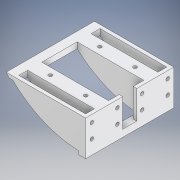
# Autodesk Inventor part: SJ004
Saved by Autodesk Inventor 2017 SP1 (Build 210196100, 196)
## iProperties
Created: 2017-06-03
Part Number: SJ004
Material: ABS Plastic
Document SubType Name: Modeling
Designer: Zach
Density: 1.06 g/cm^3
Appearance: CR White
Author: Zach
Autodesk Inventor part; units mm, degrees
ref_plane "YZ Plane" through (0, 0, 0) normal (1, 0, 0) x (0, 1, 0)
ref_plane "XZ Plane" through (0, 0, 0) normal (0, 1, 0) x (-1, 0, 0)
ref_plane "XY Plane" through (0, 0, 0) normal (0, 0, 1) x (1, 0, 0)
sketch "Sketch3" plane through (0, 0, 0) normal (0, 0, 1) x (1, 0, 0)
  circle A0 centre (0, 130) radius 130 construction
  line L0 (0, 0) -> (0, 10)
  circle A1 centre (0, 130) radius 120 construction
  line L1 (0, 0) -> (0, 50) construction
  line L2 (0, 50) -> (-102.4695, 50) construction
  arc A2 (-102.4695, 50) -> (0, 0) centre (0, 130) ccw
  arc A3 (-89.4427, 50) -> (0, 10) centre (0, 130) ccw
  line L3 (-102.4695, 50) -> (-89.4427, 50)
  dimension "d11" = 260
  dimension "d12" = 10
  dimension "d13" = 10
  dimension "d14" = 50
  constraints: 8 end point, 6 point on circle, 3 centre point, 2 vertical, 1 collinear, 1 concentric, 1 perpendicular, 1 point on line, 1 vertical alignment, 4 other
  measures "d11" diameter of A0
  measures "d12" distance of L0.start L0.end
  measures "d14" distance of L0.start L1.end
extrude "Extrusion2" add sketch "Sketch3" along normal blind 125
sketch "Sketch11" plane through (0, 0, 125) normal (0, 0, 1) x (1, 0, 0)
  line L0 (0, 0) -> (10, 0)
  line L1 (10, 0) -> (10, 10)
  line L2 (10, 10) -> (0, 10)
  line L3 (0, 10) -> (0, 0)
  dimension "d53" = 10
  dimension "d54" = 10
  constraints: 8 end point, 2 parallel, 1 horizontal, 1 perpendicular
  measures "d53" distance of L2.end L1.end
  measures "d54" distance of L1.end L0.end
extrude "Extrusion9" add sketch "Sketch11" against normal blind 125
sketch "Sketch12" plane through (10, 0, 125) normal (1, 0, 0) x (0, 0, -1)
  line L0 (0, 50) -> (0, 0) projected
  line L1 (125, 50) -> (0, 50) projected
  line L2 (0, 0) -> (125, 0)
  line L3 (125, 0) -> (125, 50)
  line L4 (125, 50) -> (0, 50)
  line L5 (0, 50) -> (0, 0)
  constraints: 8 end point, 2 parallel, 1 horizontal, 1 perpendicular
extrude "Extrusion10" add sketch "Sketch12" against normal blind 5
sketch "Sketch13" plane through (0, 0, 125) normal (0, 0, 1) x (1, 0, 0)
  line L0 (5, 10) -> (0, 10) projected
  arc A0 (-89.4427, 50) -> (0, 10) centre (0, 130) ccw projected
  line L1 (-89.4427, 50) -> (-102.4695, 50) projected
  arc A1 (-102.4695, 50) -> (0, 0) centre (0, 130) ccw projected
  line L2 (0, 0) -> (10, 0) projected
  line L3 (10, 0) -> (10, 50) projected
  line L4 (10, 50) -> (5, 50) projected
  line L5 (5, 10) -> (5, 50) projected
  line L6 (-89.4427, 50) -> (-102.4695, 50) projected
  line L7 (-102.4695, 50) -> (10, 50)
  line L8 (10, 0) -> (10, 50) projected
  line L9 (0, 0) -> (10, 0) projected
  line L10 (10, 0) -> (0, 0)
  arc A2 (-102.4695, 50) -> (0, 0) centre (0, 130) ccw
  line L11 (10, 50) -> (10, 0)
  constraints: 6 end point, 3 collinear, 2 point on circle, 1 centre point, 1 concentric
extrude "Extrusion11" add sketch "Sketch13" against normal blind 5 contours L0 A0 L7 L5
sketch "Sketch14" plane through (0, 0, 0) normal (0, 0, -1) x (-1, 0, 0)
  arc A0 (0, 0) -> (102.4695, 50) centre (0, 130) ccw projected
  line L0 (89.4427, 50) -> (102.4695, 50) projected
  arc A1 (0, 10) -> (89.4427, 50) centre (0, 130) ccw projected
  line L1 (-5, 50) -> (89.4427, 50)
  line L2 (-10, 50) -> (102.4695, 50) projected
  line L3 (-5, 10) -> (-5, 50) projected
  line L4 (-5, 10) -> (-5, 50)
  line L5 (0, 10) -> (-5, 10) projected
  line L6 (-5, 10) -> (0, 10)
  arc A2 (0, 10) -> (89.4427, 50) centre (0, 130) ccw projected
  arc A3 (0, 10) -> (89.4427, 50) centre (0, 130) ccw
  line L7 (-10, 0) -> (0, 0) projected
  line L8 (0, 10) -> (-5, 10) projected
  line L9 (-5, 50) -> (-5, 10) projected
  line L10 (-10, 50) -> (-5, 50) projected
  line L11 (-10, 0) -> (-10, 50) projected
  constraints: 6 end point, 3 collinear, 2 point on circle, 1 centre point, 1 concentric
extrude "Extrusion12" add sketch "Sketch14" against normal blind 5 contours A1 L5 L3 L1
sketch "Sketch15" plane through (10, 50, 125) normal (1, 0, 0) x (0, 0, -1)
  line L0 (0, -50) -> (0, 0) construction
  line L1 (0, -50) -> (125, -50) construction
  line L2 (0, 0) -> (20, 0) construction
  line L3 (20, 0) -> (20, -50) construction
  line L4 (20, -50) -> (0, -50) construction
  line L5 (0, -50) -> (0, 0) construction
  line L6 (125, 0) -> (0, 0) construction
  line L7 (37.5, 0) -> (52.5, 0) construction
  line L8 (52.5, 0) -> (52.5, -50) construction
  line L9 (52.5, -50) -> (37.5, -50) construction
  line L10 (37.5, -50) -> (37.5, 0) construction
  line L11 (72.5, 0) -> (87.5, 0) construction
  line L12 (87.5, 0) -> (87.5, -50) construction
  line L13 (87.5, -50) -> (72.5, -50) construction
  line L14 (72.5, -50) -> (72.5, 0) construction
  line L15 (125, -50) -> (125, 0) construction
  line L16 (125, 0) -> (105, 0) construction
  line L17 (105, 0) -> (105, -50) construction
  line L18 (105, -50) -> (125, -50) construction
  line L19 (125, -50) -> (125, 0) construction
  circle A0 centre (8.75, -10) radius 2.5
  circle A1 centre (8.75, -30) radius 2.5
  circle A2 centre (45, -10) radius 2.5
  circle A3 centre (45, -30) radius 2.5
  circle A4 centre (80, -10) radius 2.5
  circle A5 centre (80, -30) radius 2.5
  circle A6 centre (116.25, -10) radius 2.5
  circle A7 centre (116.25, -30) radius 2.5
  dimension "d63" = 20
  dimension "d64" = 15
  dimension "d65" = 20
  dimension "d66" = 15
  dimension "d69" = 5
  dimension "d70" = 5
  dimension "d71" = 5
  dimension "d72" = 5
  dimension "d73" = 5
  dimension "d74" = 5
  dimension "d75" = 5
  dimension "d76" = 5
  dimension "d77" = 8.75
  dimension "d78" = 8.75
  dimension "d79" = 7.5
  dimension "d80" = 7.5
  dimension "d81" = 10
  dimension "d82" = 20
  dimension "d114" = 36.25
  dimension "d115" = 36.25
  constraints: 32 end point, 8 centre point, 8 parallel, 6 horizontal alignment, 6 point on line, 4 horizontal, 4 perpendicular, 4 vertical alignment
  measures "d63" distance of L3.end L4.end
  measures "d64" distance of L12.end L13.end
  measures "d65" distance of L18.end L17.end
  measures "d66" distance between parallel lines of L8 L10
  measures "d69" diameter of A0
  measures "d70" diameter of A1
  measures "d71" diameter of A2
  measures "d72" diameter of A3
  measures "d73" diameter of A4
  measures "d74" diameter of A5
  measures "d75" diameter of A6
  measures "d76" diameter of A7
  measures "d77" distance from line of L19 A6.centre
  measures "d78" distance from line of L0 A0.centre
  measures "d79" distance from line of L10 A2.centre
  measures "d80" distance from line of L14 A4.centre
  measures "d81" distance from line of L6 A0.centre
  measures "d82" distance of A0.centre A1.centre
  measures "d114" distance of A2.centre A0.centre
  measures "d115" distance of A6.centre A4.centre
extrude "Extrusion13" cut sketch "Sketch15" against normal blind 5
sketch "Sketch16" plane through (-102.4695, 50, 125) normal (0, 1, 0) x (1, 0, 0)
  line L0 (112.4695, 125) -> (112.4695, 0) projected
  line L1 (0, 125) -> (0, 0) projected
  line L2 (112.4695, 107.5) -> (0, 107.5)
  line L3 (0, 107.5) -> (0, 87.5)
  line L4 (0, 87.5) -> (112.4695, 87.5)
  line L5 (112.4695, 87.5) -> (112.4695, 107.5)
  line L6 (112.4695, 37.5) -> (0, 37.5)
  line L7 (0, 37.5) -> (0, 17.5)
  line L8 (0, 17.5) -> (112.4695, 17.5)
  line L9 (112.4695, 17.5) -> (112.4695, 37.5)
  line L10 (112.4695, 125) -> (0, 125) projected
  line L11 (0, 0) -> (102.4695, 0) projected
  point P0 (102.4695, 125)
  dimension "d85" = 20
  dimension "d87" = 20
  dimension "d88" = 17.5
  dimension "d89" = 17.5
  constraints: 16 end point, 4 parallel, 4 point on line, 2 horizontal, 2 perpendicular
  measures "d85" distance of L3.end L2.end
  measures "d87" distance of L7.end L6.end
  measures "d88" distance between parallel lines of L10 L2
  measures "d89" distance between parallel lines of L11 L8
extrude "Extrusion14" add sketch "Sketch16" against normal blind 50 contours L0 L4 L1 L2 | L0 L8 L1 L6
sketch "Sketch19" plane through (10, 0, 125) normal (1, 0, 0) x (0, 0, -1)
  line L0 (52.5, 50) -> (72.5, 50)
  line L1 (72.5, 50) -> (72.5, 10)
  line L2 (72.5, 10) -> (52.5, 10)
  line L3 (52.5, 10) -> (52.5, 50)
  line L4 (0, 0) -> (0, 50) projected
  line L5 (125, 50) -> (0, 50) projected
  point P0 (125, 0)
  dimension "d95" = 20
  dimension "d96" = 52.5
  dimension "d97" = 40
  constraints: 8 end point, 2 parallel, 1 horizontal, 1 horizontal alignment, 1 perpendicular, 1 point on line
  measures "d95" distance between parallel lines of L1 L3
  measures "d96" distance between parallel lines of L4 L3
  measures "d97" distance of L2.end L0.start
extrude "Extrusion16" cut sketch "Sketch19" against normal blind 5
sketch "Sketch20" plane through (0, 0, 0) normal (0, 0, -1) x (-1, 0, 0)
  line L0 (0, 0) -> (-10, 0) projected
  arc A0 (0, 0) -> (102.4695, 50) centre (-4.8387, 139.9164) ccw
  line L1 (102.4695, 0) -> (0, 0) projected
  line L2 (0, 0) -> (102.4695, 0)
  line L3 (102.4695, 50) -> (102.4695, 0) projected
  line L4 (102.4695, 0) -> (102.4695, 50)
  line L5 (102.4695, 50) -> (102.4695, 0)
  dimension "d100" = 140
  constraints: 6 end point, 2 collinear, 2 point on circle, 1 centre point, 1 perpendicular
  measures "d100" radius of A0
extrude "Extrusion17" cut sketch "Sketch20" against normal through all
sketch "Sketch21" plane through (-102.4695, 50, 125) normal (0, 1, 0) x (1, 0, 0)
  circle A0 centre (85, 27.5) radius 2.5
  circle A1 centre (35, 27.5) radius 2.5
  circle A2 centre (85, 97.5) radius 2.5
  circle A3 centre (35, 97.5) radius 2.5
  line L0 (102.4695, 17.5) -> (102.4695, 5) projected
  line L1 (13.0268, 17.5) -> (107.4695, 17.5) projected
  line L2 (13.0268, 87.5) -> (107.4695, 87.5) projected
  line L3 (0, 125) -> (0, 0) projected
  dimension "d103" = 5
  dimension "d104" = 5
  dimension "d105" = 5
  dimension "d106" = 5
  dimension "d108" = 50
  dimension "d109" = 10
  dimension "d110" = 10
  dimension "d113" = 35
  constraints: 4 centre point, 2 horizontal alignment, 2 vertical alignment
  measures "d103" diameter of A0
  measures "d104" diameter of A1
  measures "d105" diameter of A2
  measures "d106" diameter of A3
  measures "d108" distance of A0.centre A1.centre
  measures "d109" distance from line of L1 A0.centre
  measures "d110" distance from line of L2 A2.centre
  measures "d113" distance from line of L3 A1.centre
extrude "Extrusion18" cut sketch "Sketch21" against normal through all
sketch "Sketch23" plane through (0, 0, 125) normal (0, 0, 1) x (1, 0, 0)
  line L0 (0, 0) -> (0, 5)
  arc A0 (-98.0733, 45) -> (0, 0) centre (4.8387, 139.9164) ccw
  line L1 (-98.0733, 45) -> (-93.0733, 45)
  arc A1 (-93.0733, 45) -> (0, 5) centre (4.9972, 144.9108) ccw
  arc A2 (-102.4695, 50) -> (0, 0) centre (4.8387, 139.9164) ccw projected
  dimension "d118" = 5
  dimension "d119" = 5
  dimension "d120" = 5
  dimension "d122" = 140
  dimension "d123" = 140
  constraints: 5 point on circle, 4 end point, 2 centre point, 1 horizontal, 1 vertical
  measures "d118" distance of L0.start L0.end
  measures "d119" vertical distance of A2.start L1.start
  measures "d120" distance of L1.start L1.end
  measures "d122" radius of A0
  measures "d123" radius of A1
extrude "Extrusion20" cut sketch "Sketch23" against normal through all
sketch "Sketch24" plane through (-89.4427, 50, 87.5) normal (0, 1, 0) x (1, 0, 0)
  line L0 (0, 82.5) -> (0, 70) projected
  line L1 (89.4427, -37.5) -> (89.4427, 87.5) projected
  line L2 (0, 82.5) -> (89.4427, 82.5)
  line L3 (89.4427, 82.5) -> (89.4427, 69.85)
  line L4 (89.4427, 69.85) -> (0, 69.85)
  line L5 (0, 69.85) -> (0, 82.5)
  line L6 (94.4427, 0) -> (0, 0) projected
  line L7 (89.4427, 50) -> (89.4427, 0) projected
  line L8 (0, 0) -> (89.4427, 0)
  line L9 (89.4427, 0) -> (89.4427, 50)
  line L10 (89.4427, 50) -> (0, 50)
  line L11 (0, 50) -> (0, 0)
  line L12 (0, -32.5) -> (94.4427, -32.5) projected
  line L13 (94.4427, -20) -> (89.4427, -20) projected
  line L14 (0, -32.5) -> (89.4427, -32.5)
  line L15 (89.4427, -32.5) -> (89.4427, -20)
  line L16 (89.4427, -20) -> (0, -20)
  line L17 (0, -20) -> (0, -32.5)
  constraints: 24 end point, 6 parallel, 3 horizontal, 3 perpendicular, 1 point on line
extrude "Extrusion21" cut sketch "Sketch24" against normal through all
body "Solid2"
